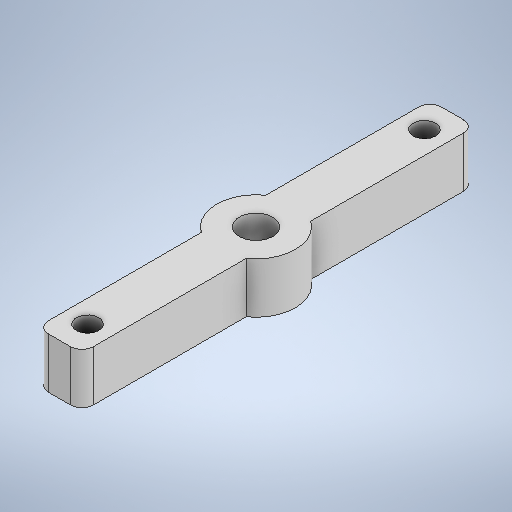
# Autodesk Inventor part: tmp1
Saved by Autodesk Inventor 2025.2 (Build 292293000, 293)
## iProperties
Created: 2025-03-20
Part Number: tmp1
Material: 一般
Document SubType Name: Modeling
Designer: mahhy
Density: 1 g/cm^3
Appearance: 既定
Author: mahhy
## iProperties of the stored document tmp1_3D プリント.ipt
Created: 2025-03-20
Part Number: tmp1_3D プリント
Material: 一般
Document SubType Name: Modeling
Designer: mahhy
Density: 1 g/cm^3
Appearance: 既定
Author: mahhy
Autodesk Inventor part; units mm, degrees
ref_plane "YZ Plane" through (0, 0, 0) normal (1, 0, 0) x (0, 1, 0)
ref_plane "XZ Plane" through (0, 0, 0) normal (0, 1, 0) x (-1, 0, 0)
ref_plane "XY Plane" through (0, 0, 0) normal (0, 0, 1) x (1, 0, 0)
sketch "スケッチ1" plane through (0, 0, 0) normal (0, 1, 0) x (-1, 0, 0)
  line L0 (-2, 17.5) -> (2, 17.5)
  line L1 (2, 17.5) -> (2, -17.5)
  line L2 (2, -17.5) -> (-2, -17.5)
  line L3 (-2, -17.5) -> (-2, 17.5)
  circle A0 centre (0, 0) radius 3.5
  point P0 (0, 17.5)
  point P1 (0, -17.5)
  point P2 (2, 0)
  point P3 (2, -2.8723)
  point P4 (2, 2.8723)
  point P5 (-2, 2.8723)
  point P6 (-2, -2.8723)
  dimension "d0" = 4
  dimension "d1" = 35
  dimension "d2" = 7
  constraints: 8 end point, 3 midpoint, 2 parallel, 1 centre point, 1 coincident, 1 horizontal, 1 horizontal alignment, 1 perpendicular, 1 vertical alignment
  measures "d0" distance of L1.end L2.end
  measures "d1" distance of L0.end L1.end
  measures "d2" diameter of A0
extrude "押し出し1" add sketch "スケッチ1" along normal blind 4.5
sketch "スケッチ2" plane through (0, 4.5, 0) normal (0, 1, 0) x (1, 0, 0)
  point P0 (0, 0)
hole "穴1" at (0, 4.5, 0) direction (0, -1, 0) diameter 3 depth 8
sketch "スケッチ3" plane through (0, 4.5, 0) normal (0, 1, 0) x (1, 0, 0)
  line L0 (0, -15) -> (0, 15)
  point P0 (0, 0)
  point P1 (0, 0)
  dimension "d12" = 30
  constraints: 2 coincident, 2 end point, 1 midpoint, 1 vertical
  measures "d12" distance of L0.start L0.end
hole "穴2" at (0, 4.5, -15) at (0, 4.5, 15) direction (0, -1, 0) diameter 2 depth 8
fillet "フィレット1" radius 1 4 edges at (2, 2.25, 17.5) (-2, 2.25, 17.5) (2, 2.25, -17.5) (-2, 2.25, -17.5)
